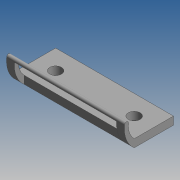
# Autodesk Inventor part: P051_HautGrenouillere
Saved by Autodesk Inventor 2021.3 (Build 253353000, 353)
## iProperties
Created: 2022-01-14
Part Number: P051_HautGrenouillere
Material: Générique
Document SubType Name: Modeling
Designer: gabri
Density: 1 g/cm^3
Appearance: Par défaut
Author: gabri
Autodesk Inventor part; units mm, degrees
ref_plane "YZ Plane" through (0, 0, 0) normal (1, 0, 0) x (0, 1, 0)
ref_plane "XZ Plane" through (0, 0, 0) normal (0, 1, 0) x (-1, 0, 0)
ref_plane "XY Plane" through (0, 0, 0) normal (0, 0, 1) x (1, 0, 0)
sketch "Sketch2" plane through (0, 0, 0) normal (0, 0, 1) x (1, 0, 0)
  line L0 (15, -5) -> (-15, -5)
  line L1 (-15, -5) -> (-15, 5)
  line L2 (-15, 5) -> (15, 5)
  line L3 (15, 5) -> (15, -5)
  line L4 (15, -5) -> (-15, 5) construction
  line L5 (-15, -5) -> (15, 5) construction
  circle A0 centre (-10, 0) radius 1.5
  circle A1 centre (10, 0) radius 1.5
  line L6 (-21, 0) -> (21, 0) construction
  point P0 (0, 0)
  point P1 (0, 0)
  dimension "d0" = 30
  dimension "d1" = 10
  dimension "d2" = 3
  dimension "d3" = 3
  dimension "d4" = 20
  dimension "d5" = 5
  constraints: 12 end point, 3 midpoint, 2 centre point, 2 parallel, 2 point on line, 1 horizontal, 1 perpendicular
  measures "d0" distance of L1.end L2.end
  measures "d1" distance between parallel lines of L0 L2
  measures "d2" diameter of A0
  measures "d3" diameter of A1
  measures "d4" distance of A1.centre A0.centre
  measures "d5" distance from line of L3 A1.centre
extrude "Extrusion1" add sketch "Sketch2" along normal blind 2
sketch "Sketch3" plane through (15, -5, 0) normal (1, 0, 0) x (0, 0, -1)
  line L0 (0, 0) -> (0, 10) construction
  line L1 (0, 10) -> (-2, 10) construction
  line L2 (-2, 0) -> (-2, 10) construction
  line L3 (0, 0) -> (-2, 0) construction
  arc A0 (-6.1418, -2.4651) -> (0, 0) centre (-5.4133, 4.6034) ccw
  arc A1 (-6.1913, -1.4792) -> (-2, 0) centre (-5.6284, 3.6034) ccw
  arc A2 (-6.1913, -1.4792) -> (-6.1418, -2.4651) centre (-6.2463, -1.9762) ccw
  line L4 (-2, 0) -> (0, 0)
  line L5 (1.7196, 5) -> (-8.1858, 5) construction
  point P0 (0, 5)
  dimension "d8" = 1
  dimension "d9" = 0.5
  dimension "d10" = 0.3966
  dimension "d11" = 1.3966
  dimension "d12" = 3.6284
  dimension "d13" = 3.4133
  dimension "d14" = 6.9762
  constraints: 6 point on circle, 3 centre point, 2 end point, 1 collinear, 1 tangent
  measures "d8" vertical distance of A1.centre A0.centre
  measures "d9" radius of A2
  measures "d10" distance from line of L5 A0.centre
  measures "d11" distance from line of L5 A1.centre
  measures "d12" distance from line of L2 A1.centre
  measures "d13" distance from line of L2 A0.centre
  measures "d14" distance from line of L5 A2.centre
extrude "Extrusion2" add sketch "Sketch3" against normal blind 2
sketch "Sketch4" plane through (-15, -5, 0) normal (-1, 0, 0) x (0, 0, 1)
  arc A0 (0, 0) -> (6.1418, -2.4651) centre (5.4133, 4.6034) ccw construction
  arc A1 (6.1418, -2.4651) -> (6.1913, -1.4792) centre (6.2463, -1.9762) ccw construction
  arc A2 (2, 0) -> (6.1913, -1.4792) centre (5.6284, 3.6034) ccw construction
  line L0 (0, 0) -> (2, 0) construction
  line L1 (0, 0) -> (2, 0)
  arc A3 (2, 0) -> (6.1913, -1.4792) centre (5.6284, 3.6034) ccw
  arc A4 (0, 0) -> (6.1418, -2.4651) centre (5.4133, 4.6034) ccw
  arc A5 (6.1418, -2.4651) -> (6.1913, -1.4792) centre (6.2463, -1.9762) ccw
  point P0 (0, 5)
  constraints: 6 point on circle, 4 concentric, 3 centre point, 2 end point, 1 collinear
extrude "Extrusion3" add sketch "Sketch4" against normal blind 2
sketch "Sketch5" plane through (13, -5, 0) normal (-1, 0, 0) x (0, 0, 1)
  arc A0 (6.1418, -2.4651) -> (6.1913, -1.4792) centre (6.2463, -1.9762) ccw construction
  circle A1 centre (6.2463, -1.9762) radius 0.5
  point P0 (0, 5)
  constraints: 1 centre point, 1 coincident, 1 concentric
extrude "Extrusion4" add sketch "Sketch5" along normal up to surface (26 mm away)
body "Solid1"
